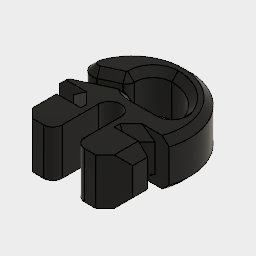
cable_clip_round (Autodesk Fusion 360 design; units mm, degrees)
Autodesk Fusion 360 part; units mm, degrees
note: some values were not read from the file. Set by a fixed rule: which sketch regions a step uses.
sketch "base" plane through (0, 0, 0) normal (0, 0, 1) x (1, 0, 0)
  line L0 (-3.4, 0) -> (-2.2, 0)
  arc A0 (-2.2, 0) -> (-1.2, 1) centre (-2.2, 1) ccw
  line L1 (-1.2, 1) -> (-1.2, 4.9)
  line L2 (-3.4, 0) -> (-5.4, 2)
  line L3 (-5.4, 3.6) -> (-2.8, 3.6)
  line L4 (-2.8, 3.8) -> (-4.4, 5.4)
  line L5 (-2.2, 0) -> (0, 0) construction
  line L6 (-5.4, 3.6) -> (-5.4, 2)
  line L7 (-4.4, 5.4) -> (-5.9, 5.4)
  arc A1 (0, 13.5) -> (-5.9, 5.4) centre (0, 7.3012) ccw
  line L8 (0, 13.5) -> (0, 0) construction
  line L9 (-2.8, 3.8) -> (-2.8, 3.6)
  arc A2 (0, 6.1) -> (-1.2, 4.9) centre (0, 4.9) ccw
  arc A3 (0, 11.6) -> (0, 7.6) centre (0, 9.6) ccw
  line L10 (-1.8689, 7.9805) -> (-5.2649, 6.3969)
  arc A4 (-5.2649, 6.3969) -> (-5.9, 5.4) centre (-4.8, 5.4) ccw
  line L11 (-4.3723, 7.9165) -> (-2.4611, 8.8077)
  arc A5 (-2.4611, 8.8077) -> (-1.9994, 9.552) centre (-2.7992, 9.5328) ccw
  arc A6 (-5.8807, 9.2613) -> (-4.3723, 7.9165) centre (-4.8372, 8.9135) ccw
  arc A7 (-1.0934, 7.9253) -> (-1.8689, 7.9805) centre (-1.5308, 7.2555) ccw
  line L12 (4.4, 5.4) -> (5.9, 5.4)
  line L13 (2.8, 3.8) -> (4.4, 5.4)
  line L14 (2.8, 3.8) -> (2.8, 3.6)
  line L15 (5.4, 3.6) -> (2.8, 3.6)
  line L16 (5.4, 3.6) -> (5.4, 2)
  line L17 (3.4, 0) -> (5.4, 2)
  line L18 (3.4, 0) -> (2.2, 0)
  arc A8 (1.2, 1) -> (2.2, 0) centre (2.2, 1) ccw
  arc A9 (1.2, 4.9) -> (0, 6.1) centre (0, 4.9) ccw
  line L19 (1.2, 1) -> (1.2, 4.9)
  arc A10 (5.9, 5.4) -> (0, 13.5) centre (0, 7.3012) ccw
  line L20 (3.0323, 7.6) -> (0, 7.6)
  arc A11 (3.9516, 8.9937) -> (0, 11.6) centre (0, 7.3012) ccw
  arc A12 (3.0323, 7.6) -> (3.9516, 8.9937) centre (3.0323, 8.6) ccw
  dimension "d6" = 4.2
  dimension "d7" = 135
  dimension "d8" = 45
  dimension "d9" = 1
  dimension "d10" = 1.2
  dimension "d27" = 0.2
  dimension "d28" = 2.6
  dimension "d29" = 1.6
  dimension "d31" = 2
  dimension "d32" = 1.8
  dimension "d60" = 1.5
  dimension "d63" = 2
  dimension "d64" = 1.5
  dimension "d65" = 1.9
  dimension "d66" = 0.7
  dimension "d70" = 1.1
  dimension "d71" = 1
  dimension "d73" = 25
  dimension "d74" = 0.8
  dimension "d75" = 1.1
  dimension "d76" = 0.8
  dimension "d78" = 1.9
  dimension "d79" = 1
  measures "d6" distance of A0.end L6
  measures "d7" angle of L0 L2
  measures "d8" angle of L3 L4
  measures "d9" radius of A0
  measures "d10" distance of L5.end L1
  measures "d27" distance of L4.start L3.end
  measures "d28" distance of L6 L3.end
  measures "d29" distance of L2.end L3.start
  measures "d31" distance of L0.start L2.end
  measures "d32" distance of L3.start L7
  measures "d60" distance of L4.end L7.end
  measures "d63" radius of A3
  measures "d64" distance of A2.start A3.end
  measures "d65" distance of A1.start A3.start
  measures "d66" distance of L4.end A2.start
  measures "d70" radius of A4
  measures "d71" distance of L10 L11
  measures "d73" angle of L7 L10
  measures "d74" radius of A7
  measures "d75" radius of A6
  measures "d76" radius of A5
  measures "d78" distance of A10 A11
  measures "d79" radius of A12
extrude "Extrude1" add sketch "base" along normal blind 5 contours L0 A0 L1 L2 L3 L4 L6 L7 A1 L9 A2 A3 L10 A4 L11 A5 A6 A7 L12 L13 L14 L15 L16 L17 L18 A8 A9 L19 A10 L20 A11 A12
chamfer "Chamfer1" distance 1 angle 45 12 edges at (-5.4, 2.8, 5) (-5.4, 2.8, 0) (5.4, 2.8, 5) (5.4, 2.8, 0) (-3.6, 4.6, 5) (-2.8, 3.7, 5) (2.8, 3.7, 5) (3.6, 4.6, 5) (-3.6, 4.6, 0) (-2.8, 3.7, 0) (3.6, 4.6, 0) (2.8, 3.7, 0)
chamfer "Chamfer3" distance 0.7 angle 45 24 edges at (-0.5704, 7.6831, 5) (-1.4311, 10.9971, 5) (-0.5704, 7.6831, 0) (-1.4311, 10.9971, 0) (-1.474, 8.0535, 5) (-3.5669, 7.1887, 5) (-1.474, 8.0535, 0) (-3.5669, 7.1887, 0) (-3.4167, 8.3621, 5) (-2.1194, 9.1111, 5) (-3.4167, 8.3621, 0) (-2.1194, 9.1111, 0) (-5.5691, 8.0924, 5) (-5.5691, 8.0924, 0) (1.9307, 13.1917, 5) (1.9307, 13.1917, 0) (-5.7277, 5.991, 5) (-5.7277, 5.991, 0) (1.5162, 7.6, 5) (3.8671, 8.0494, 5) (2.3668, 10.8898, 5) (2.3668, 10.8898, 0) (3.8671, 8.0494, 0) (1.5162, 7.6, 0)
equation "d65 = d78"
